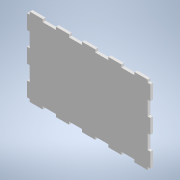
# Autodesk Inventor part: bottom
Saved by Autodesk Inventor 2020 (Build 240168000, 168)
## iProperties
Created: 2022-02-14
Part Number: bottom
Material: Generic
Document SubType Name: Modeling
Designer: rwte
Density: 1 g/cm^3
Appearance: Default
Author: rwte
Autodesk Inventor part; units mm, degrees
ref_plane "YZ Plane" through (0, 0, 0) normal (1, 0, 0) x (0, 1, 0)
ref_plane "XZ Plane" through (0, 0, 0) normal (0, 1, 0) x (-1, 0, 0)
ref_plane "XY Plane" through (0, 0, 0) normal (0, 0, 1) x (1, 0, 0)
sketch "Sketch1" plane through (0, 0, 0) normal (0, 0, 1) x (1, 0, 0)
  line L0 (-65.5, -40.5) -> (65.5, -40.5)
  line L1 (65.5, -40.5) -> (65.5, 40.5)
  line L2 (65.5, 40.5) -> (-65.5, 40.5)
  line L3 (-65.5, 40.5) -> (-65.5, -40.5)
  line L4 (-65.5, -40.5) -> (65.5, 40.5) construction
  line L5 (65.5, -40.5) -> (-65.5, 40.5) construction
  point P0 (0, 0)
  dimension "d0" = 131
  dimension "d1" = 81
  constraints: 12 end point, 2 midpoint, 2 parallel, 1 horizontal, 1 perpendicular
  measures "d0" distance of L0.start L0.end
  measures "d1" distance of L0.end L1.end
extrude "Extrusion1" add sketch "Sketch1" along normal blind 3
sketch "Sketch2" plane through (0, 0, 3) normal (0, 0, 1) x (1, 0, 0)
  line L0 (65.5, -40.5) -> (65.5, 40.5) projected
  line L1 (65.5, 40.5) -> (65.5, 24.3)
  line L2 (65.5, 24.3) -> (68.5, 24.3)
  line L3 (68.5, 24.3) -> (68.5, 40.5)
  line L4 (68.5, 40.5) -> (65.5, 40.5)
  line L5 (65.5, 8.1) -> (65.5, -8.1)
  line L6 (65.5, -8.1) -> (68.5, -8.1)
  line L7 (68.5, -8.1) -> (68.5, 8.1)
  line L8 (68.5, 8.1) -> (65.5, 8.1)
  line L9 (65.5, -24.3) -> (65.5, -40.5)
  line L10 (65.5, -40.5) -> (68.5, -40.5)
  line L11 (68.5, -40.5) -> (68.5, -24.3)
  line L12 (68.5, -24.3) -> (65.5, -24.3)
  line L13 (0, -60.9) -> (0, 60.9) projected
  line L14 (-91.7, 0) -> (91.7, 0) projected
  line L15 (-65.5, -40.5) -> (-65.5, 40.5)
  line L16 (-65.5, 40.5) -> (-65.5, 24.3)
  line L17 (-65.5, 24.3) -> (-68.5, 24.3)
  line L18 (-68.5, 24.3) -> (-68.5, 40.5)
  line L19 (-68.5, 40.5) -> (-65.5, 40.5)
  line L20 (-65.5, 8.1) -> (-65.5, -8.1)
  line L21 (-65.5, -8.1) -> (-68.5, -8.1)
  line L22 (-68.5, -8.1) -> (-68.5, 8.1)
  line L23 (-68.5, 8.1) -> (-65.5, 8.1)
  line L24 (-65.5, -24.3) -> (-65.5, -40.5)
  line L25 (-65.5, -40.5) -> (-68.5, -40.5)
  line L26 (-68.5, -40.5) -> (-68.5, -24.3)
  line L27 (-68.5, -24.3) -> (-65.5, -24.3)
  line L28 (65.5, 40.5) -> (-65.5, 40.5) projected
  line L29 (65.5, 40.5) -> (50.9444, 40.5)
  line L30 (50.9444, 40.5) -> (50.9444, 43.5)
  line L31 (50.9444, 43.5) -> (65.5, 43.5)
  line L32 (65.5, 43.5) -> (65.5, 40.5)
  line L33 (36.3889, 40.5) -> (21.8333, 40.5)
  line L34 (21.8333, 40.5) -> (21.8333, 43.5)
  line L35 (21.8333, 43.5) -> (36.3889, 43.5)
  line L36 (36.3889, 43.5) -> (36.3889, 40.5)
  line L37 (7.2778, 40.5) -> (-7.2778, 40.5)
  line L38 (-7.2778, 40.5) -> (-7.2778, 43.5)
  line L39 (-7.2778, 43.5) -> (7.2778, 43.5)
  line L40 (7.2778, 43.5) -> (7.2778, 40.5)
  line L41 (-21.8333, 40.5) -> (-36.3889, 40.5)
  line L42 (-36.3889, 40.5) -> (-36.3889, 43.5)
  line L43 (-36.3889, 43.5) -> (-21.8333, 43.5)
  line L44 (-21.8333, 43.5) -> (-21.8333, 40.5)
  line L45 (-50.9444, 40.5) -> (-65.5, 40.5)
  line L46 (-65.5, 40.5) -> (-65.5, 43.5)
  line L47 (-65.5, 43.5) -> (-50.9444, 43.5)
  line L48 (-50.9444, 43.5) -> (-50.9444, 40.5)
  line L49 (-68.5, -40.5) -> (-65.5, -40.5)
  line L50 (65.5, -40.5) -> (-65.5, -40.5)
  line L51 (65.5, -40.5) -> (50.9444, -40.5)
  line L52 (50.9444, -40.5) -> (50.9444, -43.5)
  line L53 (50.9444, -43.5) -> (65.5, -43.5)
  line L54 (65.5, -43.5) -> (65.5, -40.5)
  line L55 (36.3889, -40.5) -> (21.8333, -40.5)
  line L56 (36.3889, -43.5) -> (36.3889, -40.5)
  line L57 (21.8333, -43.5) -> (36.3889, -43.5)
  line L58 (21.8333, -40.5) -> (21.8333, -43.5)
  line L59 (7.2778, -40.5) -> (-7.2778, -40.5)
  line L60 (7.2778, -43.5) -> (7.2778, -40.5)
  line L61 (-7.2778, -43.5) -> (7.2778, -43.5)
  line L62 (-7.2778, -40.5) -> (-7.2778, -43.5)
  line L63 (-21.8333, -40.5) -> (-36.3889, -40.5)
  line L64 (-21.8333, -43.5) -> (-21.8333, -40.5)
  line L65 (-36.3889, -43.5) -> (-21.8333, -43.5)
  line L66 (-36.3889, -40.5) -> (-36.3889, -43.5)
  line L67 (-50.9444, -40.5) -> (-65.5, -40.5)
  line L68 (-50.9444, -43.5) -> (-50.9444, -40.5)
  line L69 (-65.5, -43.5) -> (-50.9444, -43.5)
  line L70 (-65.5, -40.5) -> (-65.5, -43.5)
  point P0 (0, 0)
  point P1 (65.5, 0)
  point P2 (65.5, -32.4)
  point P3 (65.5, 0)
  point P4 (-65.5, 0)
  point P5 (-65.5, -32.4)
  point P6 (-65.5, 0)
  point P7 (0, 43.5)
  point P8 (0, 40.5)
  point P9 (0, -43.5)
  point P10 (0, -40.5)
  point P11 (-21.8333, -40.5)
  point P12 (7.2778, -40.5)
  point P13 (-7.2778, -40.5)
  point P14 (-7.2778, 40.5)
  point P15 (7.2778, 40.5)
  point P16 (-65.5, 8.1)
  point P17 (-21.8333, 40.5)
  dimension "d4" = 3
  dimension "d5" = 16.2
  dimension "d6" = 3
  dimension "d7" = 16.2
  dimension "d10" = 3
  dimension "d11" = 16.2
  dimension "d14" = 3
  dimension "d15" = 14.5556
  dimension "d16" = 3
  dimension "d17" = 14.5556
  dimension "d21" = 3
  dimension "d22" = 14.5556
  dimension "d26" = 3
  dimension "d27" = 14.5556
  dimension "d31" = 3
  dimension "d32" = 14.5556
  dimension "d36" = 14.5556
  dimension "d37" = 14.5556
  constraints: 134 end point, 35 symmetric about line, 16 parallel, 8 perpendicular, 8 point on line, 7 midpoint, 2 horizontal alignment, 2 vertical alignment, 1 vertical
  measures "d4" distance of L1.end L2.end
  measures "d5" distance of L2.end L3.end
  measures "d6" distance of L5.end L6.end
  measures "d7" distance of L6.end L7.end
  measures "d10" distance of L0.start L10.end
  measures "d11" distance of L10.end L11.end
  measures "d14" distance of L31.end L0.end
  measures "d15" distance of L30.end L31.end
  measures "d16" distance of L36.start L33.start
  measures "d17" distance of L35.start L36.start
  measures "d21" distance of L40.start L37.start
  measures "d22" distance of L39.start L40.start
  measures "d26" distance of L44.start L41.start
  measures "d27" distance of L43.start L44.start
  measures "d31" distance of L48.start L45.start
  measures "d32" distance of L47.start L48.start
  measures "d36" distance between parallel lines of L30 L36
  measures "d37" distance from line of L44.start L38
extrude "Extrusion2" add sketch "Sketch2" against normal up to surface (3 mm away) contours L0 L12 L11 L10 | L54 L53 L52 L50 | L0 L14 L7 L6 | L56 L57 L58 L50 | L0 L8 L7 L14 | L60 L61 L13 L50 | L0 L4 L3 L2 | L13 L61 L62 L50 | L28 L38 L39 L13 | L13 L39 L40 L28 | L15 L21 L22 L14 | L14 L22 L23 L15 | L28 L30 L31 L32 | L64 L65 L66 L50 | L34 L35 L36 L28 | L28 L42 L43 L44 | L15 L25 L26 L27 | L17 L18 L19 L15 | L50 L68 L69 L70 | L46 L47 L48 L28
equation "\"d4\" = d2"
equation "\"d5\" = 0.2 * d1"
equation "\"d6\" = d8"
equation "\"d7\" = 0.2 * d9"
equation "\"d10\" = d12"
equation "\"d11\" = 0.2 * d13"
equation "\"d14\" = d4"
equation "\"d15\" = 0.111111 * d0"
equation "\"d16\" = d18"
equation "\"d17\" = d15"
equation "\"d21\" = d23"
equation "\"d22\" = d15"
equation "\"d26\" = d28"
equation "\"d27\" = d15"
equation "\"d31\" = d33"
equation "\"d32\" = d15"
equation "\"d36\" = d15"
equation "\"d37\" = d15"
equation "\"d8\" = d2"
equation "\"d9\" = d1"
equation "\"d12\" = d2"
equation "\"d13\" = d1"
equation "\"d18\" = d20"
equation "\"d20\" = d2"
equation "\"d23\" = d25"
equation "\"d25\" = d2"
equation "\"d28\" = d30"
equation "\"d30\" = d2"
equation "\"d33\" = d35"
equation "\"d35\" = d2"
equation "\"d2\" = 3"
body "Solid1"
